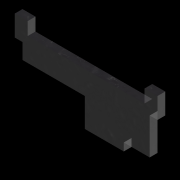
# Autodesk Inventor part: SideBottomNM
Saved by Autodesk Inventor 2019 (Build 230136000, 136)
## iProperties
Created: 2019-05-08
Part Number: SideBottomNM
Material: Acrylic, Clear
Document SubType Name: Modeling
Designer: super pig
Density: 1.19 g/cm^3
Appearance: Transparent - Clear
Mass: 2.66322 g
Surface Area: 19.78 cm^2
Volume: 2.238 cm^3
Name: Bottom Cover
Author: super pig
Autodesk Inventor part; units mm, degrees
ref_plane "YZ Plane" through (0, 0, 0) normal (1, 0, 0) x (0, 1, 0)
ref_plane "XZ Plane" through (0, 0, 0) normal (0, 1, 0) x (-1, 0, 0)
ref_plane "XY Plane" through (0, 0, 0) normal (0, 0, 1) x (1, 0, 0)
sketch "Sketch1" plane through (0, 0, 0) normal (0, 0, 1) x (1, 0, 0)
  line L0 (39, 0) -> (25, 0) projected
  line L1 (25, 0) -> (24, 0) projected
  line L2 (24, 11) -> (24, 0) projected
  line L3 (16.5, 11) -> (24, 11) projected
  line L4 (-3, 11) -> (16.5, 11) projected
  line L5 (0, 17) -> (0, 25)
  line L6 (49, 25) -> (49, 17) projected
  line L7 (49, 17) -> (52, 17) projected
  line L8 (52, 25) -> (52, 17) projected
  line L9 (49, 25) -> (52, 25) projected
  line L10 (49, 17) -> (49, 0) projected
  line L11 (39, 3) -> (49, 3) projected
  line L12 (39, 0) -> (39, 3) projected
  line L13 (0, 17) -> (0, 11)
  line L14 (2, 22) -> (2, 25)
  line L15 (2, 25) -> (0, 25)
  line L16 (0, 25) -> (0, 20)
  line L17 (47, 22) -> (47, 25)
  line L18 (47, 25) -> (49, 25)
  line L19 (0, 17) -> (0, 25) projected
  line L20 (0, 25) -> (-3, 25) projected
  line L21 (-3, 17) -> (-3, 25) projected
  line L22 (0, 17) -> (-3, 17) projected
  line L23 (2, 22) -> (47, 22)
  point P0 (0, 0)
  dimension "d2" = 5
  dimension "d4" = 5
  dimension "d5" = 3
  constraints: 16 end point, 2 horizontal, 2 point on line, 1 parallel, 1 perpendicular, 1 other
  measures "d2" distance between parallel lines of L8 L17
  measures "d4" distance between parallel lines of L14 L21
  measures "d5" distance between parallel lines of L15 L23
extrude "Extrusion1" add sketch "Sketch1" along normal blind 3
body "Solid1"
